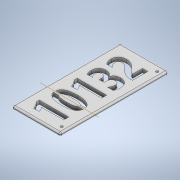
# Autodesk Inventor part: Vehicle Registration Plate V2
Saved by Autodesk Inventor 2020 (Build 240168000, 168)
## iProperties
Created: 2020-01-23
Part Number: Vehicle Registration Plate V2
Material: Generic
Document SubType Name: Modeling
Designer: maple
Density: 1 g/cm^3
Appearance: Default
Author: maple
Autodesk Inventor part; units mm, degrees
ref_plane "YZ Plane" through (0, 0, 0) normal (1, 0, 0) x (0, 1, 0)
ref_plane "XZ Plane" through (0, 0, 0) normal (0, 1, 0) x (-1, 0, 0)
ref_plane "XY Plane" through (0, 0, 0) normal (0, 0, 1) x (1, 0, 0)
sketch "Sketch1" plane through (0, 0, 0) normal (0, 1, 0) x (-1, 0, 0)
  line L0 (0, 0) -> (-101.6, 0)
  line L1 (-101.6, 0) -> (-101.6, -228.6)
  line L2 (-101.6, -228.6) -> (0, -228.6)
  line L3 (0, -228.6) -> (0, 0)
  dimension "d0" = 101.6
  dimension "d1" = 228.6
  constraints: 8 end point, 2 parallel, 1 horizontal, 1 perpendicular
  measures "d0" distance of L2.end L1.end
  measures "d1" distance of L1.end L0.end
extrude "Extrusion1" add sketch "Sketch1" along normal blind 7.62
sketch "Sketch2" plane through (0, 7.62, 0) normal (0, 1, 0) x (1, 0, 0)
  line L0 (0, 228.6) -> (0, 0) projected
  line L1 (0, 114.3) -> (101.6, 114.3)
  line L2 (101.6, 0) -> (101.6, 228.6) projected
  line L3 (0, 0) -> (101.6, 0) projected
  line L4 (50.8, 0) -> (50.8, 228.6)
  line L5 (101.6, 228.6) -> (0, 228.6) projected
  line L6 (101.6, 0) -> (101.6, 228.6) projected
  line L7 (101.6, 228.6) -> (0, 228.6) projected
  line L8 (0, 228.6) -> (0, 0) projected
  line L9 (0, 0) -> (101.6, 0) projected
  line L10 (11.0143, -52.7017) -> (11.0143, 281.0593) construction
  line L11 (11.0143, 281.0593) -> (90.4253, 281.0593) construction
  line L12 (90.4253, 281.0593) -> (90.4253, -52.7017) construction
  line L13 (90.4253, -52.7017) -> (11.0143, -52.7017) construction
  line L14 (19.024, 38.3911) -> (81.3412, 38.3911)
  line L15 (81.3412, 38.3911) -> (81.3412, 27.7034)
  line L16 (81.3412, 27.7034) -> (34.1226, 27.7034)
  spline S0 degree 2 poles (34.1226, 27.7034) (35.1405, 26.7986) (36.837, 24.3669) (38.2507, 21.6526) (39.2686, 18.7686) (39.4383, 17.2983) knots 0 0 0 1 2 3 4 4 4
  line L17 (39.4383, 17.2983) -> (28.1284, 17.2983)
  spline S1 degree 2 poles (28.1284, 17.2983) (26.6016, 21.4829) (21.8515, 28.8909) (19.024, 31.888) knots 0 0 0 1 2 2 2
  line L18 (19.024, 31.888) -> (19.024, 38.3911)
  spline S2 degree 2 poles (82.4156, 69.889) (82.4156, 52.4719) (51.8225, 52.4719) knots 0 0 0 1 1 1
  spline S3 degree 2 poles (51.8225, 52.4719) (35.9888, 52.4719) (19.3633, 61.9156) (19.3633, 70.8504) knots 0 0 0 1 2 2 2
  spline S4 degree 2 poles (19.3633, 70.8504) (19.3633, 87.8717) (50.4088, 87.8717) knots 0 0 0 1 1 1
  spline S5 degree 2 poles (50.4088, 87.8717) (65.9033, 87.8717) (82.4156, 78.5976) (82.4156, 69.889) knots 0 0 0 1 2 2 2
  spline S6 degree 2 poles (29.5987, 70.398) (29.5987, 63.3859) (51.4832, 63.3859) knots 0 0 0 1 1 1
  spline S7 degree 2 poles (51.4832, 63.3859) (72.1237, 63.3859) (72.1237, 70.2283) knots 0 0 0 1 1 1
  spline S8 degree 2 poles (72.1237, 70.2283) (72.1237, 76.9011) (50.8612, 76.9011) knots 0 0 0 1 1 1
  spline S9 degree 2 poles (50.8612, 76.9011) (29.5987, 76.9011) (29.5987, 70.398) knots 0 0 0 1 1 1
  line L19 (19.024, 118.4648) -> (81.3412, 118.4648)
  line L20 (81.3412, 118.4648) -> (81.3412, 107.777)
  line L21 (81.3412, 107.777) -> (34.1226, 107.777)
  spline S10 degree 2 poles (34.1226, 107.777) (35.1405, 106.8722) (36.837, 104.4406) (38.2507, 101.7262) (39.2686, 98.8422) (39.4383, 97.3719) knots 0 0 0 1 2 3 4 4 4
  line L22 (39.4383, 97.3719) -> (28.1284, 97.3719)
  spline S11 degree 2 poles (28.1284, 97.3719) (26.6016, 101.5566) (21.8515, 108.9645) (19.024, 111.9616) knots 0 0 0 1 2 2 2
  line L23 (19.024, 111.9616) -> (19.024, 118.4648)
  line L24 (79.362, 134.1854) -> (67.6563, 134.1854)
  spline S12 degree 2 poles (67.6563, 134.1854) (72.1237, 139.1052) (72.1237, 145.6084) knots 0 0 0 1 1 1
  spline S13 degree 2 poles (72.1237, 145.6084) (72.1237, 149.7365) (67.7128, 154.3169) (63.7544, 154.3169) knots 0 0 0 1 2 2 2
  spline S14 degree 2 poles (63.7544, 154.3169) (59.6263, 154.3169) (55.2155, 148.662) (55.2155, 143.6857) knots 0 0 0 1 2 2 2
  line L25 (55.2155, 143.6857) -> (55.2155, 139.1618)
  line L26 (55.2155, 139.1618) -> (44.9235, 139.1618)
  line L27 (44.9235, 139.1618) -> (44.9235, 143.3464)
  spline S15 degree 2 poles (44.9235, 143.3464) (44.9235, 152.8467) (37.0066, 152.8467) knots 0 0 0 1 1 1
  spline S16 degree 2 poles (37.0066, 152.8467) (29.5987, 152.8467) (29.5987, 145.5518) knots 0 0 0 1 1 1
  spline S17 degree 2 poles (29.5987, 145.5518) (29.5987, 140.6886) (33.5571, 136.0516) knots 0 0 0 1 1 1
  line L28 (33.5571, 136.0516) -> (22.5866, 136.0516)
  spline S18 degree 2 poles (22.5866, 136.0516) (19.3633, 141.1975) (19.3633, 147.9834) knots 0 0 0 1 1 1
  spline S19 degree 2 poles (19.3633, 147.9834) (19.3633, 155.5045) (27.7891, 163.8172) (34.4619, 163.8172) knots 0 0 0 1 2 2 2
  spline S20 degree 2 poles (34.4619, 163.8172) (46.4504, 163.8172) (49.4475, 154.1473) knots 0 0 0 1 1 1
  line L29 (49.4475, 154.1473) -> (49.6737, 154.1473)
  spline S21 degree 2 poles (49.6737, 154.1473) (50.4653, 159.2933) (58.2691, 165.2875) (63.924, 165.2875) knots 0 0 0 1 2 2 2
  spline S22 degree 2 poles (63.924, 165.2875) (72.463, 165.2875) (82.4156, 155.2783) (82.4156, 146.4566) knots 0 0 0 1 2 2 2
  spline S23 degree 2 poles (82.4156, 146.4566) (82.4156, 138.9356) (79.362, 134.1854) knots 0 0 0 1 1 1
  line L30 (70.201, 184.8535) -> (70.201, 205.4939)
  line L31 (70.201, 205.4939) -> (81.3412, 205.4939)
  line L32 (81.3412, 205.4939) -> (81.3412, 173.0913)
  line L33 (81.3412, 173.0913) -> (76.7607, 173.0913)
  spline S24 degree 2 poles (76.7607, 173.0913) (72.0671, 173.0913) (64.6026, 175.5794) (58.7215, 179.4248) (54.141, 183.9487) (52.3315, 185.9845) knots 0 0 0 1 2 3 4 4 4
  spline S25 degree 2 poles (52.3315, 185.9845) (50.4088, 188.1333) (46.9593, 191.3566) (43.5098, 193.5621) (39.9472, 194.6365) (37.968, 194.6365) knots 0 0 0 1 2 3 4 4 4
  spline S26 degree 2 poles (37.968, 194.6365) (34.0661, 194.6365) (30.0511, 191.0739) (30.0511, 187.4547) knots 0 0 0 1 2 2 2
  spline S27 degree 2 poles (30.0511, 187.4547) (30.0511, 181.1778) (36.3281, 175.4098) knots 0 0 0 1 1 1
  line L34 (36.3281, 175.4098) -> (24.5093, 175.4098)
  spline S28 degree 2 poles (24.5093, 175.4098) (19.3633, 181.7998) (19.3633, 189.7733) knots 0 0 0 1 1 1
  spline S29 degree 2 poles (19.3633, 189.7733) (19.3633, 193.5055) (21.7949, 199.3866) (26.2623, 203.4582) (32.7089, 205.607) (36.6674, 205.607) knots 0 0 0 1 2 3 4 4 4
  spline S30 degree 2 poles (36.6674, 205.607) (40.852, 205.607) (47.4117, 203.5147) (52.7839, 200.0652) (57.2512, 195.5978) (59.287, 193.1662) knots 0 0 0 1 2 3 4 4 4
  spline S31 degree 2 poles (59.287, 193.1662) (60.7573, 191.5263) (63.5848, 188.5292) (66.3557, 186.2107) (69.0135, 184.8535) (70.201, 184.8535) knots 0 0 0 1 2 3 4 4 4
  point P0 (50.8, 114.3)
  constraints: 5 midpoint, 4 end point, 2 other
emboss "Emboss1" sketch "Sketch2" operation cut depth 7.62 direction (0, -1, 0) contours L23 L19 L4 L1 | L1 L4 L21 S10 L22 S11 L23 | S30 S31 L30 L31 L32 L33 S24 S25 L4 | L4 S25 S26 S27 L34 S28 S29 S30 | L4 L19 L20 L1 | L1 L20 L21 L4 | L16 S0 L17 S1 L18 L14 L4 | L4 L14 L15 L16 | S21 S22 S23 L24 S12 S13 S14 L25 L26 L4 | L4 L26 L27 S15 S16 S17 L28 S18 S19 S20 L29 S21 | S5 S2 S3 L4 S6 S7 S8 S9 | L4 S9 S6 S3 S4 S5
sketch "Sketch7" plane through (0, 7.62, 0) normal (0, 1, 0) x (1, 0, 0)
  line L0 (72.1237, 70.2283) -> (86.6151, 70.2283)
  line L1 (86.6151, 70.2283) -> (86.6151, 67.6883)
  line L2 (86.6151, 67.6883) -> (15.875, 67.6883)
  line L3 (15.875, 67.6883) -> (15.875, 72.7683)
  line L4 (15.875, 72.7683) -> (86.6151, 72.7683)
  line L5 (86.6151, 72.7683) -> (86.6151, 67.6883)
  point P0 (0, 0)
  dimension "d6" = 2.54
  dimension "d7" = 5.08
  constraints: 12 end point, 2 horizontal, 2 parallel, 2 perpendicular
  measures "d6" distance of L0.end L1.end
  measures "d7" distance of L2.end L3.end
extrude "Extrusion2" add sketch "Sketch7" against normal blind 7.62
fillet "Fillet1" radius 3.175 12 edges at (0, 0, -114.3) (0, 7.62, -114.3) (0, 3.81, -228.6) (50.8, 0, -228.6) (50.8, 7.62, -228.6) (101.6, 3.81, -228.6) (101.6, 7.62, -114.3) (101.6, 0, -114.3) (50.8, 0, 0) (50.8, 7.62, 0) (101.6, 3.81, 0) (0, 3.81, 0)
sketch "Sketch9" plane through (0, 7.62, 0) normal (0, 1, 0) x (1, 0, 0)
  line L0 (101.6, 225.425) -> (101.6, 3.175) projected
  line L1 (101.6, 3.175) -> (91.44, 3.175)
  line L2 (3.175, 3.175) -> (98.425, 3.175) projected
  line L3 (91.44, 3.175) -> (91.44, 13.335)
  line L4 (101.6, 225.425) -> (91.44, 225.425)
  line L5 (91.44, 225.425) -> (91.44, 215.265)
  circle A0 centre (91.44, 13.335) radius 2.54
  circle A1 centre (91.44, 215.265) radius 2.54
  point P0 (0, 0)
  dimension "d17" = 10.16
  dimension "d18" = 10.16
  dimension "d19" = 10.16
  dimension "d20" = 10.16
  dimension "d21" = 5.08
  dimension "d22" = 5.08
  constraints: 8 end point, 2 centre point, 2 coincident, 2 perpendicular, 1 horizontal, 1 point on line
  measures "d17" distance of L0.end L1.end
  measures "d18" distance of L1.end L3.end
  measures "d19" distance of L0.start L4.end
  measures "d20" distance of L4.end L5.end
  measures "d21" diameter of A0
  measures "d22" diameter of A1
extrude "Extrusion4" cut sketch "Sketch9" against normal blind 7.62
body "Solid1"
